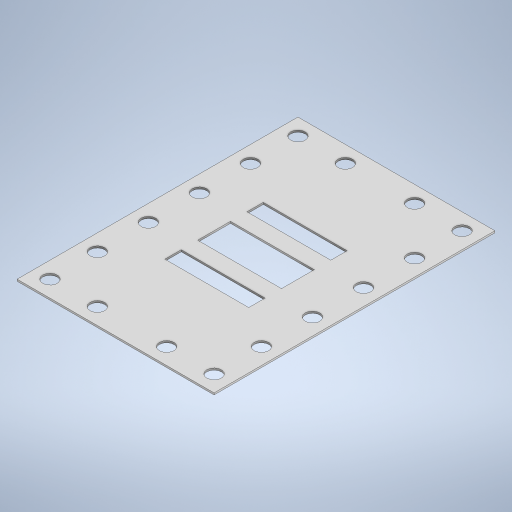
# Autodesk Inventor part: 1-33
Saved by Autodesk Inventor 2024.2 (Build 282272000, 272)
## iProperties
Created: 2024-11-02
Part Number: 1-33
Material: Generic
Document SubType Name: Modeling
Designer: Jimena Brenes
Density: 1 g/cm^3
Appearance: Default
Author: Jimena Brenes
Autodesk Inventor part; units mm, degrees
ref_plane "YZ Plane" through (0, 0, 0) normal (1, 0, 0) x (0, 1, 0)
ref_plane "XZ Plane" through (0, 0, 0) normal (0, 1, 0) x (-1, 0, 0)
ref_plane "XY Plane" through (0, 0, 0) normal (0, 0, 1) x (1, 0, 0)
sketch "Sketch1" plane through (0, 0, 0) normal (0, 1, 0) x (-1, 0, 0)
  line L0 (0, 0) -> (-54, 0)
  line L1 (-54, 0) -> (-54, -77)
  line L2 (-54, -77) -> (0, -77)
  line L3 (0, -77) -> (0, 0)
  line L4 (-4.5, -4.5) -> (-49.5, -4.5) construction
  line L5 (-49.5, -4.5) -> (-49.5, -72.5) construction
  line L6 (-49.5, -72.5) -> (-4.5, -72.5) construction
  line L7 (-4.5, -72.5) -> (-4.5, -4.5) construction
  circle A0 centre (-4.5, -4.5) radius 2
  circle A1 centre (-17.5, -4.5) radius 2
  circle A2 centre (-49.5, -4.5) radius 2
  circle A3 centre (-49.5, -17.5) radius 2
  circle A4 centre (-49.5, -31.5) radius 2
  circle A5 centre (-49.5, -45.5) radius 2
  circle A6 centre (-49.5, -59.5) radius 2
  circle A7 centre (-49.5, -72.5) radius 2
  circle A8 centre (-36.5, -72.5) radius 2
  circle A9 centre (-17.5, -72.5) radius 2
  circle A10 centre (-4.5, -72.5) radius 2
  circle A11 centre (-4.5, -59.5) radius 2
  circle A12 centre (-4.5, -45.5) radius 2
  circle A13 centre (-4.5, -31.5) radius 2
  circle A14 centre (-4.5, -17.5) radius 2
  circle A15 centre (-36.5, -4.5) radius 2
  dimension "d0" = 54
  dimension "d1" = 77
  dimension "d2" = 4
  dimension "d3" = 4
  dimension "d5" = 4
  dimension "d6" = 4
  dimension "d7" = 4
  dimension "d8" = 4
  dimension "d9" = 4
  dimension "d10" = 4
  dimension "d11" = 4
  dimension "d12" = 4
  dimension "d13" = 4
  dimension "d14" = 4
  dimension "d15" = 4
  dimension "d16" = 4
  dimension "d17" = 4
  dimension "d18" = 4.5
  dimension "d20" = 4.5
  dimension "d21" = 4.5
  dimension "d22" = 4.5
  dimension "d23" = 13
  dimension "d27" = 14
  dimension "d28" = 14
  dimension "d29" = 14
  dimension "d30" = 4.5
  dimension "d31" = 4
  dimension "d32" = 13
  dimension "d33" = 19
  dimension "d34" = 13
  dimension "d35" = 14
  dimension "d36" = 14
  dimension "d37" = 14
  dimension "d38" = 13
  dimension "d39" = 19
  constraints: 16 centre point, 16 end point, 12 point on line, 4 coincident, 4 parallel, 2 horizontal, 2 perpendicular
  measures "d0" distance of L0.start L0.end
  measures "d1" distance between parallel lines of L2 L0
  measures "d2" diameter of A0
  measures "d3" diameter of A1
  measures "d5" diameter of A2
  measures "d6" diameter of A3
  measures "d7" diameter of A4
  measures "d8" diameter of A5
  measures "d9" diameter of A6
  measures "d10" diameter of A7
  measures "d11" diameter of A8
  measures "d12" diameter of A9
  measures "d13" diameter of A10
  measures "d14" diameter of A11
  measures "d15" diameter of A12
  measures "d16" diameter of A13
  measures "d17" diameter of A14
  measures "d18" distance between parallel lines of L0 L4
  measures "d20" distance from line of L2 L5.end
  measures "d21" distance from line of L2 L6.end
  measures "d22" distance between parallel lines of L3 L7
  measures "d23" distance of A3.centre L4.end
  measures "d27" distance of A3.centre A4.centre
  measures "d28" distance of A5.centre A4.centre
  measures "d29" distance of A6.centre A5.centre
  measures "d30" distance between parallel lines of L1 L5
  measures "d31" diameter of A15
  measures "d32" distance of L4.end A15.centre
  measures "d33" distance of A1.centre A15.centre
  measures "d34" distance of L4.start A14.centre
  measures "d35" distance of A13.centre A14.centre
  measures "d36" distance of A12.centre A13.centre
  measures "d37" distance of A12.centre A11.centre
  measures "d38" distance of L6.end A9.centre
  measures "d39" distance of A8.centre A9.centre
extrude "Extrusion1" add sketch "Sketch1" along normal blind 0.5
sketch "Sketch2" plane through (0, 0.5, 0) normal (0, 1, 0) x (1, 0, 0)
  line L0 (15.5, 47.5) -> (38.5, 47.5)
  line L1 (38.5, 47.5) -> (38.5, 52)
  line L2 (38.5, 52) -> (15.5, 52)
  line L3 (15.5, 52) -> (15.5, 47.5)
  line L4 (27, 0) -> (27, 77) construction
  line L5 (54, 0) -> (54, 77) projected
  line L6 (0, 38.5) -> (54, 38.5) construction
  line L7 (54, 77) -> (0, 77) projected
  line L8 (15.5, 34) -> (38.5, 34)
  line L9 (38.5, 34) -> (38.5, 43)
  line L10 (38.5, 43) -> (15.5, 43)
  line L11 (15.5, 43) -> (15.5, 34)
  line L12 (15.5, 25) -> (38.5, 25)
  line L13 (38.5, 25) -> (38.5, 29.5)
  line L14 (38.5, 29.5) -> (15.5, 29.5)
  line L15 (15.5, 29.5) -> (15.5, 25)
  circle A0 centre (4.5, 45.5) radius 2 projected
  circle A1 centre (4.5, 31.5) radius 2 projected
  point P0 (0, 0)
  point P1 (15.5, 38.5)
  point P2 (27, 43)
  point P3 (27, 47.5)
  point P4 (27, 29.5)
  dimension "d42" = 27
  dimension "d43" = 38.5
  dimension "d47" = 9
  dimension "d48" = 23
  dimension "d49" = 4.5
  dimension "d50" = 4.5
  dimension "d51" = 23
  dimension "d52" = 4.5
  dimension "d53" = 4.5
  constraints: 28 end point, 6 parallel, 5 midpoint, 5 point on line, 4 perpendicular, 3 horizontal, 1 vertical
  measures "d42" distance between parallel lines of L5 L4
  measures "d43" distance between parallel lines of L7 L6
  measures "d47" distance between parallel lines of L10 L8
  measures "d48" distance between parallel lines of L9 L11
  measures "d49" distance between parallel lines of L10 L0
  measures "d50" distance between parallel lines of L8 L14
  measures "d51" distance between parallel lines of L1 L3
  measures "d52" distance between parallel lines of L14 L12
  measures "d53" distance between parallel lines of L0 L2
extrude "Extrusion2" cut sketch "Sketch2" against normal through all contours L3 L2 L1 L0 | L11 L10 L9 L8 | L15 L14 L13 L12
body "Solid1"
